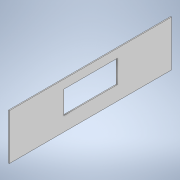
# Autodesk Inventor part: TorraumFront
Saved by Autodesk Inventor 2021 (Build 250183000, 183)
## iProperties
Created: 2022-02-22
Part Number: TorraumFront
Material: Generisch
Document SubType Name: Modeling
Designer: valen
Density: 1 g/cm^3
Appearance: Vorgabe
Author: valen
Autodesk Inventor part; units mm, degrees
ref_plane "YZ Plane" through (0, 0, 0) normal (1, 0, 0) x (0, 1, 0)
ref_plane "XZ Plane" through (0, 0, 0) normal (0, 1, 0) x (-1, 0, 0)
ref_plane "XY Plane" through (0, 0, 0) normal (0, 0, 1) x (1, 0, 0)
sketch "Skizze1" plane through (0, 0, 0) normal (1, 0, 0) x (0, 1, 0)
  line L0 (0, 0) -> (192, 0)
  line L1 (192, 0) -> (192, -680)
  line L2 (192, -680) -> (0, -680)
  line L3 (0, -680) -> (0, 0)
  line L4 (156, -228) -> (60, -228)
  line L5 (60, -228) -> (60, -452)
  line L6 (60, -452) -> (156, -452)
  line L7 (156, -452) -> (156, -228)
  dimension "d0" = 192
  dimension "d1" = 680
  dimension "d7" = 224
  dimension "d8" = 96
  dimension "d9" = 228
  dimension "d10" = 60
  constraints: 16 end point, 4 parallel, 2 horizontal, 2 perpendicular
  measures "d0" distance of L1.end L2.end
  measures "d1" distance between parallel lines of L2 L0
  measures "d7" distance between parallel lines of L6 L4
  measures "d8" distance between parallel lines of L5 L7
  measures "d9" distance between parallel lines of L0 L4
  measures "d10" distance between parallel lines of L5 L3
extrude "Extrusion2" add sketch "Skizze1" along normal blind 4
